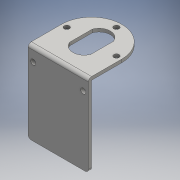
# Autodesk Inventor part: motor mount
Saved by Autodesk Inventor 2016 (Build 200138000, 138)
## iProperties
Created: 2015-09-14
Part Number: motor mount
Material: Generic
Document SubType Name: Modeling
Designer: Hulbert Office
Density: 1 g/cm^3
Appearance: Default
Author: Hulbert Office
Autodesk Inventor part; units mm, degrees
ref_plane "YZ Plane" through (0, 0, 0) normal (1, 0, 0) x (0, 1, 0)
ref_plane "XZ Plane" through (0, 0, 0) normal (0, 1, 0) x (-1, 0, 0)
ref_plane "XY Plane" through (0, 0, 0) normal (0, 0, 1) x (1, 0, 0)
sketch "Sketch1" plane through (0, 0, 0) normal (1, 0, 0) x (0, 1, 0)
  line L0 (0, 0) -> (0, 49.2)
  line L1 (0, 49.2) -> (37.6, 49.2)
  line L2 (37.6, 51.2) -> (-2, 51.2)
  line L3 (-2, 51.2) -> (-2, 0)
  line L4 (37.6, 51.2) -> (37.6, 49.2)
  line L5 (0, 0) -> (-2, 0)
  dimension "d0" = 49.2
  dimension "d1" = 37.6
  dimension "d2" = 2
  constraints: 12 end point, 3 perpendicular, 1 horizontal, 1 vertical, 1 other
  measures "d0" distance of L0.start L0.end
  measures "d1" distance of L0.end L1.end
  measures "d2" distance between parallel lines of L1 L2
extrude "Extrusion1" add sketch "Sketch1" along normal blind 37.6
fillet "Fillet1" radius 2 1 edges at (18.8, -2, 51.2)
fillet "Fillet2" radius 2 2 edges at (37.6, -1, 0) (0, -1, 0)
sketch "Sketch2" plane through (0, 37.6, 51.2) normal (0, 0, 1) x (1, 0, 0)
  line L0 (0, -39.6) -> (37.6, -39.6)
  line L1 (0, -39.6) -> (0, -18.8)
  line L2 (0, -37.6) -> (0, 0)
  circle A0 centre (18.794722, -18.794721) radius 15.5
  circle A1 centre (3.294722, -18.794721) radius 1.65
  circle A2 centre (34.3, -18.8) radius 1.65
  circle A3 centre (18.8, -3.3) radius 1.65
  circle A4 centre (18.794722, -18.794721) radius 18.805278
  line L3 (37.6, -37.6) -> (37.6, 0)
  line L4 (37.6, -18.8) -> (37.6, 0)
  line L5 (0, 0) -> (37.6, 0)
  line L6 (37.6, 0) -> (0, 0)
  line L7 (0, 0) -> (0, -18.16472)
  arc A5 (37.6, -18.8) -> (0, -18.8) centre (18.8, -18.8) ccw
  line L8 (18.8, -18.8) -> (18.8, -11.8)
  line L9 (18.8, -11.8) -> (18.8, -25.8)
  line L10 (18.8, -18.8) -> (25.4, -18.8)
  line L11 (25.4, -18.8) -> (12.2, -18.8)
  line L12 (18.8, -11.8) -> (12.2, -11.8)
  line L13 (12.2, -11.8) -> (12.2, -25.8)
  line L14 (12.2, -25.8) -> (25.4, -25.8)
  line L15 (25.4, -25.8) -> (25.4, -11.8)
  line L16 (25.4, -11.8) -> (18.8, -11.8)
  arc A6 (25.4, -11.8) -> (12.2, -11.8) centre (18.8, -14.132381) ccw
  arc A7 (12.2, -25.8) -> (25.4, -25.8) centre (18.8, -23.467619) ccw
  dimension "d8" = 31
  dimension "d7" = 20.8
  dimension "d9" = 3.3
  dimension "d10" = 3.3
  dimension "d11" = 3.3
  dimension "d16" = 7
  dimension "d17" = 14
  dimension "d18" = 6.6
  dimension "d19" = 13.2
  dimension "d20" = 7
  dimension "d21" = 7
  constraints: 26 end point, 8 point on circle, 7 centre point, 4 perpendicular, 4 point on line, 2 collinear, 1 horizontal, 1 horizontal alignment, 1 midpoint, 1 parallel, 1 tangent, 1 vertical, 2 other
  measures "d7" distance of L0.start L1.end
  measures "d9" diameter of A1
  measures "d10" diameter of A2
  measures "d11" diameter of A3
  measures "d16" distance of L8.start L8.end
  measures "d17" distance of L8.end L9.end
  measures "d18" distance of L8.start L10.end
  measures "d19" distance of L10.end L11.end
  measures "d20" radius of A6
  measures "d21" radius of A7
extrude "Extrusion2" cut sketch "Sketch2" against normal through all contours A0 A2 | A0 A2 | A3 A0 | A0 A3 | A1 A0 | A0 A1
sketch "Sketch2 outline for Extrusion3" plane through (0, 37.6, 51.2) normal (0, 0, 1) x (1, 0, 0)
  line L0 (0, 0) -> (0, -18.8)
  arc A0 (18.8, 0) -> (0, -18.8) centre (18.8, -18.8) ccw
  line L1 (18.8, 0) -> (0, 0)
  arc A1 (37.6, -18.8) -> (18.8, 0) centre (18.8, -18.8) ccw
  line L2 (37.6, 0) -> (18.8, 0)
  line L3 (37.6, -18.8) -> (37.6, 0)
extrude "Extrusion3" cut sketch "Sketch2 outline for Extrusion3" against normal through all
extrude "Extrusion4" cut sketch "Sketch2" against normal blind 37.6 contours L11 L13 L12 L8 | L10 L15 L14 L9 | L8 L16 L15 L10 | L9 L14 L13 L11 | L12 A6 L16 | L14 A7
sketch "Sketch4" plane through (0, 0, 49.2) normal (0, 1, 0) x (1, 0, 0)
  line L0 (37.6, -2) -> (0, -2) projected
  line L1 (0, -2) -> (0, 6.4)
  line L2 (0, 47.2) -> (0, 0) projected
  line L3 (18.8, -2) -> (3.2, -2)
  line L4 (3.2, -2) -> (34.4, -2)
  line L5 (3.2, -2) -> (3.2, 6.4)
  circle A0 centre (3.2, 6.4) radius 1.6
  line L6 (34.4, -2) -> (34.4, 6.4)
  circle A1 centre (34.4, 6.4) radius 1.6
  point P0 (0, 49.2)
  dimension "d24" = 8.4
  dimension "d25" = 15.6
  dimension "d26" = 31.2
  dimension "d27" = 3.2
  dimension "d28" = 3.2
  constraints: 10 end point, 3 point on line, 2 centre point, 2 coincident, 1 midpoint, 1 parallel, 1 vertical
  measures "d24" distance of L0.end L1.end
  measures "d25" distance of L3.start L3.end
  measures "d26" distance of L3.end L4.end
  measures "d27" diameter of A0
  measures "d28" diameter of A1
extrude "Extrusion5" cut sketch "Sketch4" against normal blind 37.6
body "Solid1"
